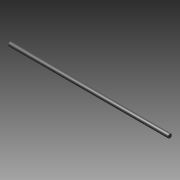
# Autodesk Inventor part: PSFG10-400
Saved by Autodesk Inventor 2014 SP1 (Build 180222100, 222)
## iProperties
Category: PARTsolutions
Company: MISUMI
Created: 2014-10-09
Part Number: PSFG10-400
Catalog Web Link: www.cadenas.de
Description: SFJ, SFU, SSFJ, SSFU, PSFJ, PSFU, PSSFJ, PSSFU, RSFJ, PSFG, PSSFG-Shafts Solid Type
Vendor: MISUMI
Document SubType Name: Modeling
Designer: PARTuser1
Manufacturer: MISUMI
Mass: 31.4083 g
Surface Area: 127.044 cm^2
Volume: 31.4083 cm^3
Density: 1 g/cm^3
Material: Generic
Appearance: PSOLRGB-175-175-175
PSOL_IDENT_0: {\\10.0.0.236\data_v8\23d-libs\misumi\metric\01_linear_shafts\sfj.prj},305 {VTYP=3D},{NB=PSFG10-400}
PSOL_IDENT_1: ,{LINA=PSFG10-400},{NN=SFJ, SFU, SSFJ, SSFU, PSFJ, PSFU, PSSFJ, PSSFU, RSFJ, PSFG, PSSFG},{DATE=26.0
PSOL_IDENT_2: 8.2014 04:38:56},{GEOMDATE=24.07.2014 04:44:00},{VERSION=},{LINEID=60},{LINESUBID=-1},{WBVAR=TS,MAT,
PSOL_IDENT_3: ST,ALT1,L,ALT3,SC,WSC,X,ALT4,FC,WFC,A,E,ALT5,RC,WRC,Y,ALT6,VC,WVC,F,ALT7,KC,G}  {NB=PSFG10-400},{LIN
PSOL_IDENT_4: A=PSFG10-400},{KT=DUMMY},{PN=PSFG10-400},{TYPE=PSFG},{TS=f8},{TSALG= 'g6','g6' , 'h5','h5' , 'f8','f
PSOL_IDENT_5: 8' },{MAT=S45C},{MATALG= 'S45C','1045 Carbon Steel' , 'SUS304','304 Stainless Steel' },{HARD=-},{ST=
PSOL_IDENT_6: HCP10},{STALG= 'HCP10','Hard Chrome Plating Plating Hardness: HV750 ~ Plating Thickness: 10 microns
PSOL_IDENT_7: or More' },{D=10},{ALT1=},{L=400.0},{LALG=[20:800/1]},{LMIN=20},{LMAX=800},{LPN=-400},{C=0.5 or Less
PSOL_IDENT_8: },{C2=0.5},{ALT3=},{ALT3ALG= '','w/o Wrench Flats' , 'SC','with SC (Wrench Flats at One Location)' ,
PSOL_IDENT_9: 'WSC','with WSC (Wrench Flats at Two Locations)' },{SC=0},{SCALG=[0]},{SCMAX=392},{WSC=0},{WSCALG=[
PSOL_IDENT_10: 0]},{WSCMAX=382},{X=0},{XALG=[0]},{XMAX=382},{WALT3=0},{LL1=0},{LL1ALG=8},{ALT3PN=},{ALT4=},{FC=0},{
PSOL_IDENT_11: FCALG=[0]},{FCMAX=30},{WFC=0},{WFCALG=[0]},{WFCMAX=30},{A=0},{AALG=[0]},{AMAX=0},{E=0},{EALG=[0]},{E
PSOL_IDENT_12: MAX=398},{HHALT4=0.0},{ALT4PN=},{ALT5=},{ALT5ALG= '','w/o 90-deg. Set Screw Flat' , 'RC','with RC (9
PSOL_IDENT_13: 0-deg. Set Screw Flat at One Location)' , 'WRC','with WRC (90-deg. Set Screw Flats at Two Locations)'
PSOL_IDENT_14: },{RC=0},{RCALG=[0]},{RCMIN=2},{RCMAX=400},{WRC=0},{WRCALG=[0]},{WRCMIN=2},{WRCMAX=396},{Y=0},{YALG=
PSOL_IDENT_15: [0]},{YMIN=2},{YMAX=398},{BB1=0},{HHALT5=0.0},{ALT5PN=},{ALT6=},{ALT6ALG= '','w/o V Groove' , 'VC','
PSOL_IDENT_16: with VC (V Groove at One Location)' , 'WVC','with WVC (V Grooves at Two Locations)' },{VC=0},{VCALG=
PSOL_IDENT_17: [0]},{VCMAX=400},{WVC=0},{WVCALG=[0]},{WVCMIN=2},{WVCMAX=400},{F=0},{FALG=[0]},{FMAX=400},{WALT6=0},
PSOL_IDENT_18: {ALT6PN=},{ALT7=},{ALT7ALG= '','Not applicable' },{KC=0},{KCALG=[0]},{KCMAX1=398},{KCMAX2=400},{G=0}
PSOL_IDENT_19: ,{GALG=[0]},{GMIN=0},{GMAX1=30},{GMAX2=30},{BB=0},{TT=0.0},{ALT7PN=},{ERRORPN=},{ERRORALT34=OK},{ERR
PSOL_IDENT_20: ORALT35=OK},{ERRORALT36=OK},{ERRORALT37=OK},{ERRORALT45=OK},{ERRORALT46=OK},{ERRORALT47=OK},{ERRORAL
PSOL_IDENT_21: T56=OK},{ERRORALT57=OK},{ERRORALT67=OK}
SUPPLIER: MISUMI
ARTICLENO: PSFG10-400
BOMINFO: PSFG10-400
CREATOR: CADENAS GmbH
Title: PSFG10-400
Author: Cadenas PARTsolutions
Comments: Shafts Solid Type
Autodesk Inventor part; units mm, degrees
ref_plane "YZ Plane" through (0, 0, 0) normal (1, 0, 0) x (0, 1, 0)
ref_plane "XZ Plane" through (0, 0, 0) normal (0, 1, 0) x (-1, 0, 0)
ref_plane "XY Plane" through (0, 0, 0) normal (0, 0, 1) x (1, 0, 0)
sketch "Sketch_3" plane through (0, 0, 0) normal (0, 0, 1) x (1, 0, 0)
  line L0 (400, 0.225) -> (20, 0.225)
  line L1 (20, 0.225) -> (20, 4.5)
  line L2 (20, 4.5) -> (20.475, 4.975)
  line L3 (20.475, 4.975) -> (399.525, 4.975)
  line L4 (399.525, 4.975) -> (400, 4.5)
  line L5 (400, 4.5) -> (400, 0.225)
  line L6 (400, 0.225) -> (20, 0.225)
  dimension "d1" = 380
  constraints: 14 end point
  measures "d1" distance of L4.end L1.end
revolve "Revolution1" add sketch "Sketch_3" angle 360 about axis through (400, 0.225, 0) along (1, 0, 0)
body "Solid1"
